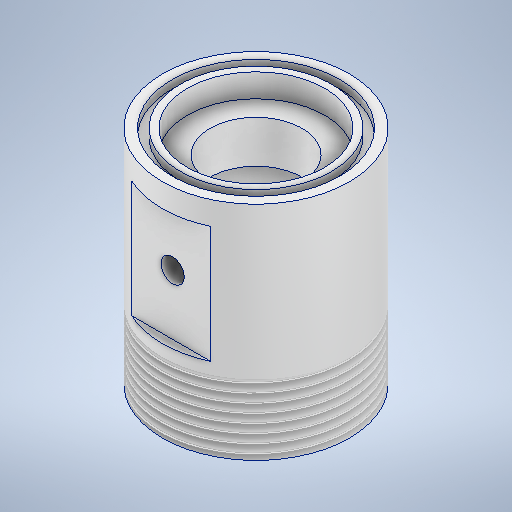
# Autodesk Inventor part: Passthrough Base Insert
Saved by Autodesk Inventor 2025 (Build 290162000, 162)
## iProperties
Created: 2024-04-16
Part Number: Passthrough Base Insert
Material: Aluminum 6061
Document SubType Name: Modeling
Designer: cfang
Density: 2.7 g/cm^3
Appearance: Aluminum - Flat
Author: cfang
Autodesk Inventor part; units mm, degrees
ref_plane "YZ Plane" through (0, 0, 0) normal (1, 0, 0) x (0, 1, 0)
ref_plane "XZ Plane" through (0, 0, 0) normal (0, 1, 0) x (-1, 0, 0)
ref_plane "XY Plane" through (0, 0, 0) normal (0, 0, 1) x (1, 0, 0)
sketch "Sketch1" plane through (0, 0, 0) normal (0, 1, 0) x (-1, 0, 0)
  circle A0 centre (0, 0) radius 16
  dimension "d0" = 32
  constraints: 1 centre point, 1 coincident
  measures "d0" diameter of A0
extrude "Extrusion1" add sketch "Sketch1" along normal blind 38
thread "Thread1" size "M32x1.5" class "6g" standard "ANSI Metric M Profile" length 12
sketch "Sketch2" plane through (0, 0, 0) normal (0, -1, 0) x (1, 0, 0)
  circle A0 centre (0, 0) radius 7.875
  dimension "d5" = 15.75
  constraints: 1 centre point, 1 coincident
  measures "d5" diameter of A0
extrude "Extrusion2" cut sketch "Sketch2" against normal through all
sketch "Sketch3" plane through (0, 38, 0) normal (0, 1, 0) x (1, 0, 0)
  circle A0 centre (0, 0) radius 11.75
  dimension "d8" = 23.5
  constraints: 1 centre point, 1 coincident
  measures "d8" diameter of A0
extrude "Extrusion3" cut sketch "Sketch3" against normal blind 4
sketch "Sketch4" plane through (0, 0, 0) normal (1, 0, 0) x (0, 1, 0)
  line L0 (0, 16) -> (38, 16) projected
  line L1 (34, 16) -> (14, 16)
  line L2 (14, 16) -> (14, 14.5)
  line L3 (14, 14.5) -> (34, 14.5)
  line L4 (34, 14.5) -> (34, 16)
  line L5 (0, -16) -> (38, -16) projected
  line L6 (34, -16) -> (14, -16)
  line L7 (14, -16) -> (14, -14.5)
  line L8 (14, -14.5) -> (34, -14.5)
  line L9 (34, -14.5) -> (34, -16)
  line L10 (38, -16) -> (38, 16) projected
  point P0 (0, 0)
  point P1 (14, 16)
  point P2 (14, -16)
  dimension "d11" = 20
  dimension "d12" = 1.5
  dimension "d13" = 1.5
  dimension "d33" = 4
  constraints: 16 end point, 4 parallel, 4 point on line, 2 horizontal, 2 perpendicular
  measures "d11" distance of L3.end L2.end
  measures "d12" distance of L2.end L1.end
  measures "d13" distance of L6.end L7.end
  measures "d33" distance between parallel lines of L10 L4
extrude "Extrusion4" cut sketch "Sketch4" along normal through all both and the other way through all
sketch "Sketch5" plane through (0, 0, 0) normal (0, 0, 1) x (1, 0, 0)
  line L0 (7.875, 0) -> (7.875, 34) projected
  line L1 (7.875, 26.75) -> (9.875, 26.75)
  line L2 (9.875, 26.75) -> (9.875, 21.75)
  line L3 (9.875, 21.75) -> (7.875, 21.75)
  line L4 (7.875, 21.75) -> (7.875, 26.75)
  line L5 (0, -5.7834) -> (0, 45.928)
  line L6 (-11.75, 38) -> (11.75, 38) projected
  point P0 (0, 0)
  point P1 (7.875, 21.75)
  dimension "d17" = 11.25
  dimension "d18" = 16.25
  dimension "d19" = 2
  constraints: 10 end point, 2 parallel, 1 horizontal, 1 perpendicular, 1 point on line, 1 vertical
  measures "d17" distance between parallel lines of L6 L1
  measures "d18" distance between parallel lines of L3 L6
  measures "d19" distance between parallel lines of L0 L2
revolve "Revolution1" cut sketch "Sketch5" angle 360 about axis through (0, -5.7834, 0) along (0, 1, 0)
sketch "Sketch6" plane through (6.7639, 34, -14.5) normal (0, 0, -1) x (-1, 0, 0)
  line L0 (-3.1111, -7.25) -> (16.6389, -7.25) projected
  line L1 (-3.1111, -12.25) -> (16.6389, -12.25) projected
  point P0 (6.7639, -34)
  point P1 (6.5383, -9.75)
  dimension "d20" = 5
  dimension "d21" = 2.5
  measures "d20" distance between parallel lines of L0 L1
  measures "d21" distance from line of L1 point (6.538, -9.75)
hole "Hole1" at (0.2255, 24.25, -14.5) direction (0, 0, 1) diameter 4 end through all
sketch "Sketch7" plane through (0, 38, 0) normal (0, 1, 0) x (1, 0, 0)
  circle A0 centre (0, 0) radius 12.95
  circle A1 centre (0, 0) radius 14.35
  circle A2 centre (0, 0) radius 11.75 projected
  dimension "d29" = 1.2
  dimension "d30" = 1.4
  constraints: 2 centre point, 2 coincident
  measures "d29" radial gap between concentric circles of A0 A2
  measures "d30" radial gap between concentric circles of A1 A0
extrude "Extrusion5" cut sketch "Sketch7" against normal blind 1.4 contours A1
equation "\"d21\" = 0.5 * d20"
body "Solid1"
